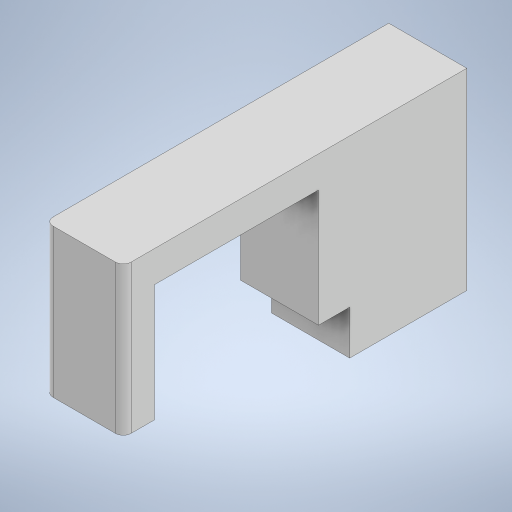
# Autodesk Inventor part: uchwyt_serwa_czlon1_pre
Saved by Autodesk Inventor 2023 (Build 270158000, 158)
## iProperties
Created: 2024-06-27
Part Number: uchwyt_serwa_czlon1_pre
Material: Ogólny
Document SubType Name: Modeling
Designer: kamil
Density: 1 g/cm^3
Appearance: Domyślna
Author: kamil
Autodesk Inventor part; units mm, degrees
ref_plane "YZ Plane" through (0, 0, 0) normal (1, 0, 0) x (0, 1, 0)
ref_plane "XZ Plane" through (0, 0, 0) normal (0, 1, 0) x (-1, 0, 0)
ref_plane "XY Plane" through (0, 0, 0) normal (0, 0, 1) x (1, 0, 0)
sketch "Szkic1" plane through (0, 0, 0) normal (1, 0, 0) x (0, 1, 0)
  line L0 (14.5, 20) -> (-14.5, 20)
  line L1 (-14.5, -20) -> (14.5, -20)
  line L2 (14.5, -20) -> (14.5, 20)
  line L3 (-14.5, 21) -> (15.5, 21)
  line L4 (15.5, 21) -> (15.5, -21)
  line L5 (15.5, -21) -> (-14.5, -21)
  line L6 (-14.5, 29) -> (23.5, 29)
  line L7 (23.5, 29) -> (23.5, -29)
  line L8 (23.5, -29) -> (-14.5, -29)
  line L9 (-14.5, 29) -> (-14.5, 21)
  line L10 (-14.5, -21) -> (-14.5, -29)
  point P0 (0, 0)
  point P1 (14.5, 0)
  point P2 (0, 20)
  dimension "d0" = 40
  dimension "d3" = 1
  dimension "d4" = 8
  dimension "d12" = 30
  dimension "d13" = 8
  constraints: 22 end point, 4 equal length, 4 vertical alignment, 3 perpendicular, 2 midpoint, 1 horizontal, 1 horizontal alignment, 1 vertical, 4 other
  measures "d0" distance of L1.start L0.end
  measures "d3" distance between parallel lines of L2 L4
  measures "d4" distance between parallel lines of L3 L6
  measures "d12" distance between parallel lines of L10 L4
  measures "d13" distance between parallel lines of L7 L4
extrude "Wyciągnięcie proste1" add sketch "Szkic1" along normal blind 20
sketch "Szkic2" plane through (20, 0, 0) normal (1, 0, 0) x (0, 0, -1)
  line L0 (29, -14.5) -> (29, 23.5) projected
  line L1 (29, -14.5) -> (29, 23.5) projected
  line L2 (29, 23.5) -> (59, 23.5)
  line L3 (59, 23.5) -> (59, -25.8001)
  line L4 (59, -25.8001) -> (29, -25.8001)
  line L5 (29, -25.8001) -> (29, 23.5)
  point P0 (0, 0)
  dimension "d7" = 30
  dimension "d8" = 49.3001
  constraints: 8 end point, 2 parallel, 1 horizontal, 1 perpendicular
  measures "d7" distance of L3.end L4.end
  measures "d8" distance between parallel lines of L4 L2
extrude "Wyciągnięcie proste2" add sketch "Szkic2" against normal up to surface (20 mm away)
fillet "Zaokrąglenie1" radius 2 2 edges at (0, 4.5, 29) (20, 4.5, 29)
